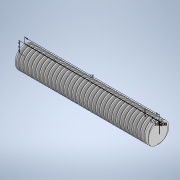
# Autodesk Inventor part: lead screw
Saved by Autodesk Inventor 2020.2 (Build 242310000, 310)
## iProperties
Created: 2021-02-15
Part Number: lead screw
Material: Generic
Document SubType Name: Modeling
Designer: Olivi
Density: 1 g/cm^3
Appearance: Default
Author: Olivi
Autodesk Inventor part; units mm, degrees
ref_plane "YZ Plane" through (0, 0, 0) normal (1, 0, 0) x (0, 1, 0)
ref_plane "XZ Plane" through (0, 0, 0) normal (0, 1, 0) x (-1, 0, 0)
ref_plane "XY Plane" through (0, 0, 0) normal (0, 0, 1) x (1, 0, 0)
sketch "Sketch2" plane through (0, 0, 0) normal (0, 0, 1) x (1, 0, 0)
  line L0 (0, 0) -> (0, 4)
  line L1 (0, 4) -> (50, 4)
  line L2 (50, 4) -> (50, 0)
  line L3 (50.9912, 4) -> (50.75, 3.1)
  line L4 (50.75, 3.1) -> (50.2412, 3.1)
  line L5 (50.2412, 3.1) -> (50, 4)
  line L6 (49.4912, 4) -> (50, 4)
  line L7 (50, 0) -> (0, 0)
  line L8 (50, 4) -> (50.9912, 4)
  dimension "d7" = 4
  dimension "d8" = 50
  dimension "d10" = 105
  dimension "d11" = 105
  dimension "d12" = 0.9
  dimension "d13" = 0
  dimension "d15" = 1.5
  dimension "d16" = 0
  constraints: 18 end point, 2 equal length, 2 parallel, 2 perpendicular, 1 collinear, 1 vertical
  measures "d7" distance of L0.start L0.end
  measures "d8" distance of L0.end L1.end
  measures "d10" angle of L4 L5
  measures "d11" angle of L4 L3
  measures "d12" distance between parallel lines of L4 L6
  measures "d13" distance between parallel lines of L6 L1
  measures "d15" distance of L3.start L6.start
  measures "d16" distance of L1.end L5.end
revolve "Revolution1" add sketch "Sketch2" angle 360 about axis through (50, 0, 0) along (-1, 0, 0) contours L0 L1 L2 L7
coil "Coil1" sketch "Sketch2" operation cut axis through (-10, 0, 0) along (-1, 0, 0) pitch 1.5 turns 100 hand right contours L8 L3 L4 L5
body "Solid2"
